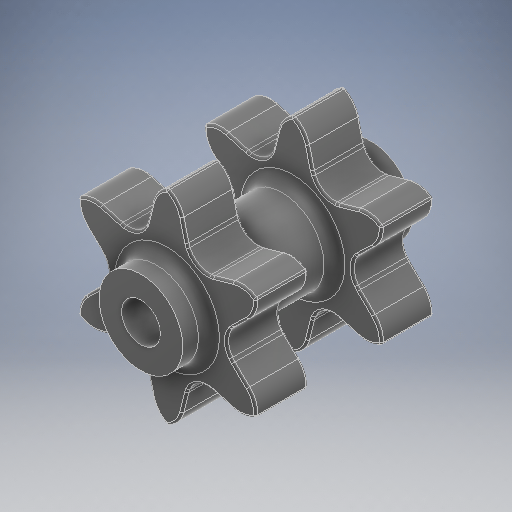
# Autodesk Inventor part: SprocketGeometry
Saved by Autodesk Inventor 2026.1 (Build 301233000, 233)
## iProperties
Created: 2025-09-26
Part Number: SprocketGeometry
Material: Plastic, Opaque Black
Document SubType Name: Modeling
Designer: Teddy
Density: 0.952 g/cm^3
Appearance: Smooth - Black
Author: Teddy
Autodesk Inventor part; units mm, degrees
ref_plane "YZ Plane" through (0, 0, 0) normal (1, 0, 0) x (0, 1, 0)
ref_plane "XZ Plane" through (0, 0, 0) normal (0, 1, 0) x (-1, 0, 0)
ref_plane "XY Plane" through (0, 0, 0) normal (0, 0, 1) x (1, 0, 0)
sketch "Sketch1" plane through (0, 0, 0) normal (0, 0, 1) x (1, 0, 0)
  line L0 (-9.7902, 3.5752) -> (-8.0084, 1.8545)
  spline S0 degree 3 poles (-10.7537, 6.0542) (-10.7758, 5.6696) (-10.7287, 5.2836) (-10.4774, 4.4609) (-10.2116, 4.004) (-9.833, 3.6171) (-9.8117, 3.596) (-9.7902, 3.5752) knots 0 0 0 0 0.414162 0.414162 0.967573 0.967573 1 1 1 1
  spline S1 degree 3 poles (-7.9913, 6.691) (-8.0201, 6.6992) (-8.049, 6.7071) (-8.5734, 6.8415) (-9.1019, 6.8432) (-9.9401, 6.6495) (-10.2979, 6.4973) (-10.6199, 6.2859) knots 0 0 0 0 0.032427 0.032427 0.585838 0.585838 1 1 1 1
  line L1 (-7.9913, 6.691) -> (-5.6103, 6.0082)
  arc A0 (-5.1715, 5.9227) -> (-2.5435, 7.44) centre (-4.8997, 8.4865) ccw
  spline S2 degree 3 poles (-10.7537, 6.0542) (-10.7533, 6.0604) (-10.7527, 6.0666) (-10.7469, 6.1132) (-10.7332, 6.1525) (-10.6948, 6.219) (-10.6676, 6.2505) (-10.6302, 6.2788) (-10.6251, 6.2824) (-10.6199, 6.2859) knots 0 0 0 0 0.066671 0.066671 0.5 0.5 0.933329 0.933329 1 1 1 1
  spline S3 degree 3 poles (-5.1715, 5.9227) (-5.1884, 5.9245) (-5.2052, 5.9265) (-5.3494, 5.9446) (-5.4802, 5.9714) (-5.6103, 6.0082) knots 0 0 0 0 0.115694 0.115694 1 1 1 1
  line L2 (-1.7989, 10.2662) -> (-2.3981, 7.8628)
  spline S4 degree 3 poles (-2.3981, 7.8628) (-2.4313, 7.7317) (-2.4735, 7.605) (-2.5299, 7.471) (-2.5366, 7.4555) (-2.5435, 7.44) knots 0 0 0 0 0.884306 0.884306 1 1 1 1
  spline S5 degree 3 poles (-0.1338, 12.34) (-0.4779, 12.1669) (-0.7886, 11.9332) (-1.3754, 11.3041) (-1.6382, 10.8456) (-1.784, 10.3242) (-1.7916, 10.2952) (-1.7989, 10.2662) knots 0 0 0 0 0.414162 0.414162 0.967573 0.967573 1 1 1 1
  spline S6 degree 3 poles (-0.1338, 12.34) (-0.1282, 12.3428) (-0.1225, 12.3454) (-0.0793, 12.3637) (-0.0384, 12.3715) (0.0384, 12.3715) (0.0793, 12.3637) (0.1225, 12.3454) (0.1282, 12.3428) (0.1338, 12.34) knots 0 0 0 0 0.066671 0.066671 0.5 0.5 0.933329 0.933329 1 1 1 1
  spline S7 degree 3 poles (1.7989, 10.2662) (1.7916, 10.2952) (1.784, 10.3242) (1.6382, 10.8456) (1.3754, 11.3041) (0.7886, 11.9332) (0.4779, 12.1669) (0.1338, 12.34) knots 0 0 0 0 0.032427 0.032427 0.585838 0.585838 1 1 1 1
  line L3 (1.7989, 10.2662) -> (2.3981, 7.8628)
  spline S8 degree 3 poles (2.5435, 7.44) (2.5366, 7.4555) (2.5299, 7.471) (2.4735, 7.605) (2.4313, 7.7317) (2.3981, 7.8628) knots 0 0 0 0 0.115694 0.115694 1 1 1 1
  arc A1 (2.5435, 7.44) -> (5.1715, 5.9227) centre (4.8997, 8.4865) ccw
  spline S9 degree 3 poles (5.6103, 6.0082) (5.4802, 5.9714) (5.3494, 5.9446) (5.2052, 5.9265) (5.1884, 5.9245) (5.1715, 5.9227) knots 0 0 0 0 0.884306 0.884306 1 1 1 1
  line L4 (7.9913, 6.691) -> (5.6103, 6.0082)
  spline S10 degree 3 poles (10.6199, 6.2859) (10.2979, 6.4973) (9.9401, 6.6495) (9.1019, 6.8432) (8.5734, 6.8415) (8.049, 6.7071) (8.0201, 6.6992) (7.9913, 6.691) knots 0 0 0 0 0.414162 0.414162 0.967573 0.967573 1 1 1 1
  spline S11 degree 3 poles (10.6199, 6.2859) (10.6251, 6.2824) (10.6302, 6.2788) (10.6676, 6.2505) (10.6948, 6.219) (10.7332, 6.1525) (10.7469, 6.1132) (10.7527, 6.0666) (10.7533, 6.0604) (10.7537, 6.0542) knots 0 0 0 0 0.066671 0.066671 0.5 0.5 0.933329 0.933329 1 1 1 1
  spline S12 degree 3 poles (9.7902, 3.5752) (9.8117, 3.596) (9.833, 3.6171) (10.2116, 4.004) (10.4774, 4.4609) (10.7287, 5.2836) (10.7758, 5.6696) (10.7537, 6.0542) knots 0 0 0 0 0.032427 0.032427 0.585838 0.585838 1 1 1 1
  line L5 (8.0084, 1.8545) -> (9.7902, 3.5752)
  spline S13 degree 3 poles (7.715, 1.5173) (7.725, 1.531) (7.7351, 1.5446) (7.8229, 1.6604) (7.9115, 1.7603) (8.0084, 1.8545) knots 0 0 0 0 0.115694 0.115694 1 1 1 1
  arc A2 (7.715, 1.5173) -> (7.715, -1.5173) centre (9.7993, 0) ccw
  spline S14 degree 3 poles (8.0084, -1.8545) (7.9115, -1.7603) (7.8229, -1.6604) (7.7351, -1.5446) (7.725, -1.531) (7.715, -1.5173) knots 0 0 0 0 0.884306 0.884306 1 1 1 1
  line L6 (9.7902, -3.5752) -> (8.0084, -1.8545)
  spline S15 degree 3 poles (10.7537, -6.0542) (10.7758, -5.6696) (10.7287, -5.2836) (10.4774, -4.4609) (10.2116, -4.004) (9.833, -3.6171) (9.8117, -3.596) (9.7902, -3.5752) knots 0 0 0 0 0.414162 0.414162 0.967573 0.967573 1 1 1 1
  spline S16 degree 3 poles (10.7537, -6.0542) (10.7533, -6.0604) (10.7527, -6.0666) (10.7469, -6.1132) (10.7332, -6.1525) (10.6948, -6.219) (10.6676, -6.2505) (10.6302, -6.2788) (10.6251, -6.2824) (10.6199, -6.2859) knots 0 0 0 0 0.066671 0.066671 0.5 0.5 0.933329 0.933329 1 1 1 1
  spline S17 degree 3 poles (7.9913, -6.691) (8.0201, -6.6992) (8.049, -6.7071) (8.5734, -6.8415) (9.1019, -6.8432) (9.9401, -6.6495) (10.2979, -6.4973) (10.6199, -6.2859) knots 0 0 0 0 0.032427 0.032427 0.585838 0.585838 1 1 1 1
  line L7 (7.9913, -6.691) -> (5.6103, -6.0082)
  spline S18 degree 3 poles (5.1715, -5.9227) (5.1884, -5.9245) (5.2052, -5.9265) (5.3494, -5.9446) (5.4802, -5.9714) (5.6103, -6.0082) knots 0 0 0 0 0.115694 0.115694 1 1 1 1
  arc A3 (5.1715, -5.9227) -> (2.5435, -7.44) centre (4.8997, -8.4865) ccw
  spline S19 degree 3 poles (2.3981, -7.8628) (2.4313, -7.7317) (2.4735, -7.605) (2.5299, -7.471) (2.5366, -7.4555) (2.5435, -7.44) knots 0 0 0 0 0.884306 0.884306 1 1 1 1
  line L8 (1.7989, -10.2662) -> (2.3981, -7.8628)
  spline S20 degree 3 poles (0.1338, -12.34) (0.4779, -12.1669) (0.7886, -11.9332) (1.3754, -11.3041) (1.6382, -10.8456) (1.784, -10.3242) (1.7916, -10.2952) (1.7989, -10.2662) knots 0 0 0 0 0.414162 0.414162 0.967573 0.967573 1 1 1 1
  spline S21 degree 3 poles (0.1338, -12.34) (0.1282, -12.3428) (0.1225, -12.3454) (0.0793, -12.3637) (0.0384, -12.3715) (-0.0384, -12.3715) (-0.0793, -12.3637) (-0.1225, -12.3454) (-0.1282, -12.3428) (-0.1338, -12.34) knots 0 0 0 0 0.066671 0.066671 0.5 0.5 0.933329 0.933329 1 1 1 1
  spline S22 degree 3 poles (-1.7989, -10.2662) (-1.7916, -10.2952) (-1.784, -10.3242) (-1.6382, -10.8456) (-1.3754, -11.3041) (-0.7886, -11.9332) (-0.4779, -12.1669) (-0.1338, -12.34) knots 0 0 0 0 0.032427 0.032427 0.585838 0.585838 1 1 1 1
  line L9 (-1.7989, -10.2662) -> (-2.3981, -7.8628)
  spline S23 degree 3 poles (-2.5435, -7.44) (-2.5366, -7.4555) (-2.5299, -7.471) (-2.4735, -7.605) (-2.4313, -7.7317) (-2.3981, -7.8628) knots 0 0 0 0 0.115694 0.115694 1 1 1 1
  arc A4 (-2.5435, -7.44) -> (-5.1715, -5.9227) centre (-4.8997, -8.4865) ccw
  spline S24 degree 3 poles (-5.6103, -6.0082) (-5.4802, -5.9714) (-5.3494, -5.9446) (-5.2052, -5.9265) (-5.1884, -5.9245) (-5.1715, -5.9227) knots 0 0 0 0 0.884306 0.884306 1 1 1 1
  line L10 (-7.9913, -6.691) -> (-5.6103, -6.0082)
  spline S25 degree 3 poles (-10.6199, -6.2859) (-10.2979, -6.4973) (-9.9401, -6.6495) (-9.1019, -6.8432) (-8.5734, -6.8415) (-8.049, -6.7071) (-8.0201, -6.6992) (-7.9913, -6.691) knots 0 0 0 0 0.414162 0.414162 0.967573 0.967573 1 1 1 1
  spline S26 degree 3 poles (-10.6199, -6.2859) (-10.6251, -6.2824) (-10.6302, -6.2788) (-10.6676, -6.2505) (-10.6948, -6.219) (-10.7332, -6.1525) (-10.7469, -6.1132) (-10.7527, -6.0666) (-10.7533, -6.0604) (-10.7537, -6.0542) knots 0 0 0 0 0.066671 0.066671 0.5 0.5 0.933329 0.933329 1 1 1 1
  spline S27 degree 3 poles (-9.7902, -3.5752) (-9.8117, -3.596) (-9.833, -3.6171) (-10.2116, -4.004) (-10.4774, -4.4609) (-10.7287, -5.2836) (-10.7758, -5.6696) (-10.7537, -6.0542) knots 0 0 0 0 0.032427 0.032427 0.585838 0.585838 1 1 1 1
  line L11 (-8.0084, -1.8545) -> (-9.7902, -3.5752)
  arc A5 (-7.715, -1.5173) -> (-7.715, 1.5173) centre (-9.7993, 0) ccw
  spline S28 degree 3 poles (-7.715, -1.5173) (-7.725, -1.531) (-7.7351, -1.5446) (-7.8229, -1.6604) (-7.9115, -1.7603) (-8.0084, -1.8545) knots 0 0 0 0 0.115694 0.115694 1 1 1 1
  spline S29 degree 3 poles (-8.0084, 1.8545) (-7.9115, 1.7603) (-7.8229, 1.6604) (-7.7351, 1.5446) (-7.725, 1.531) (-7.715, 1.5173) knots 0 0 0 0 0.884306 0.884306 1 1 1 1
  point P0 (0, 0)
extrude "Extrusion1" add sketch "Sketch1" along normal mid plane 6.35
sketch "Sketch2" plane through (0, 0, 3.175) normal (0, 0, 1) x (1, 0, 0)
  line L0 (3.048, -3.302) -> (-3.048, -3.302) construction
  line L1 (-3.302, -3.048) -> (-3.302, 3.048) construction
  line L2 (-3.048, 3.302) -> (3.048, 3.302) construction
  line L3 (3.302, 3.048) -> (3.302, -3.048) construction
  line L4 (3.302, -3.302) -> (-3.302, 3.302) construction
  line L5 (-3.302, -3.302) -> (3.302, 3.302) construction
  arc A0 (-3.302, -3.048) -> (-3.048, -3.302) centre (-3.048, -3.048) ccw construction
  arc A1 (-3.048, 3.302) -> (-3.302, 3.048) centre (-3.048, 3.048) ccw construction
  arc A2 (3.302, 3.048) -> (3.048, 3.302) centre (3.048, 3.048) ccw construction
  arc A3 (3.048, -3.302) -> (3.302, -3.048) centre (3.048, -3.048) ccw construction
  circle A4 centre (0, 0) radius 2.3495
  circle A5 centre (0, 0) radius 5.08
  dimension "d2" = 6.604
  dimension "d3" = 6.604
  dimension "d4" = 0.254
  dimension "d5" = 4.699
  dimension "d6" = 10.16
  constraints: 12 end point, 8 point on circle, 8 point on line, 8 tangent, 6 centre point, 3 equal radius, 2 coincident, 2 midpoint, 2 parallel, 1 horizontal, 1 perpendicular
  measures "d2" distance of L4.end L5.end
  measures "d3" distance of L5.end L4.start
  measures "d4" radius of A0
  measures "d5" diameter of A4
  measures "d6" diameter of A5
extrude "Extrusion2" add sketch "Sketch2" along normal blind 8.89
sketch "Sketch3" plane through (0, 0, 12.065) normal (0, 0, 1) x (1, 0, 0)
  line L0 (-9.7902, 3.5752) -> (-8.0084, 1.8545) projected
  ellipse E0 centre (-9.017, 1.1629) end of major axis (-7.5138, 0.0679) minor radius 1.1817 (-7.715, 1.5173) -> (-8.0084, 1.8545) ccw projected
  arc A0 (-7.715, -1.5173) -> (-7.715, 1.5173) centre (-9.7993, 0) ccw projected
  spline S0 degree 3 poles (-7.715, -1.5173) (-7.725, -1.531) (-7.7351, -1.5446) (-7.8229, -1.6604) (-7.9115, -1.7603) (-8.0084, -1.8545) knots 0 0 0 0 0.115694 0.115694 1 1 1 1 projected
  line L1 (-8.0084, -1.8545) -> (-9.7902, -3.5752) projected
  spline S1 degree 3 poles (-9.7902, -3.5752) (-9.8117, -3.596) (-9.833, -3.6171) (-10.2116, -4.004) (-10.4774, -4.4609) (-10.7287, -5.2836) (-10.7758, -5.6696) (-10.7537, -6.0542) knots 0 0 0 0 0.032427 0.032427 0.585838 0.585838 1 1 1 1 projected
  spline S2 degree 3 poles (-10.7537, -6.0542) (-10.7533, -6.0604) (-10.7527, -6.0666) (-10.7469, -6.1132) (-10.7332, -6.1525) (-10.6948, -6.219) (-10.6676, -6.2505) (-10.6302, -6.2788) (-10.6251, -6.2824) (-10.6199, -6.2859) knots 0 0 0 0 0.066671 0.066671 0.5 0.5 0.933329 0.933329 1 1 1 1 projected
  spline S3 degree 3 poles (-10.6199, -6.2859) (-10.2979, -6.4973) (-9.9401, -6.6495) (-9.1019, -6.8432) (-8.5734, -6.8415) (-8.049, -6.7071) (-8.0201, -6.6992) (-7.9913, -6.691) knots 0 0 0 0 0.414162 0.414162 0.967573 0.967573 1 1 1 1 projected
  line L2 (-7.9913, -6.691) -> (-5.6103, -6.0082) projected
  ellipse E1 centre (-5.5156, -7.2275) end of major axis (-3.8157, -6.4732) minor radius 1.1817 (-5.1715, -5.9227) -> (-5.6103, -6.0082) ccw projected
  arc A1 (-2.5435, -7.44) -> (-5.1715, -5.9227) centre (-4.8997, -8.4865) ccw projected
  spline S4 degree 3 poles (-2.5435, -7.44) (-2.5366, -7.4555) (-2.5299, -7.471) (-2.4735, -7.605) (-2.4313, -7.7317) (-2.3981, -7.8628) knots 0 0 0 0 0.115694 0.115694 1 1 1 1 projected
  line L3 (-2.3981, -7.8628) -> (-1.7989, -10.2662) projected
  spline S5 degree 3 poles (-1.7989, -10.2662) (-1.7916, -10.2952) (-1.784, -10.3242) (-1.6382, -10.8456) (-1.3754, -11.3041) (-0.7886, -11.9332) (-0.4779, -12.1669) (-0.1338, -12.34) knots 0 0 0 0 0.032427 0.032427 0.585838 0.585838 1 1 1 1 projected
  spline S6 degree 3 poles (-0.1338, -12.34) (-0.1282, -12.3428) (-0.1225, -12.3454) (-0.0793, -12.3637) (-0.0384, -12.3715) (0.0384, -12.3715) (0.0793, -12.3637) (0.1225, -12.3454) (0.1282, -12.3428) (0.1338, -12.34) knots 0 0 0 0 0.066671 0.066671 0.5 0.5 0.933329 0.933329 1 1 1 1 projected
  spline S7 degree 3 poles (0.1338, -12.34) (0.4779, -12.1669) (0.7886, -11.9332) (1.3754, -11.3041) (1.6382, -10.8456) (1.784, -10.3242) (1.7916, -10.2952) (1.7989, -10.2662) knots 0 0 0 0 0.414162 0.414162 0.967573 0.967573 1 1 1 1 projected
  line L4 (1.7989, -10.2662) -> (2.3981, -7.8628) projected
  ellipse E2 centre (3.5014, -8.3904) end of major axis (3.6981, -6.5411) minor radius 1.1817 (2.5435, -7.44) -> (2.3981, -7.8628) ccw projected
  arc A2 (5.1715, -5.9227) -> (2.5435, -7.44) centre (4.8997, -8.4865) ccw projected
  spline S8 degree 3 poles (5.1715, -5.9227) (5.1884, -5.9245) (5.2052, -5.9265) (5.3494, -5.9446) (5.4802, -5.9714) (5.6103, -6.0082) knots 0 0 0 0 0.115694 0.115694 1 1 1 1 projected
  line L5 (5.6103, -6.0082) -> (7.9913, -6.691) projected
  spline S9 degree 3 poles (7.9913, -6.691) (8.0201, -6.6992) (8.049, -6.7071) (8.5734, -6.8415) (9.1019, -6.8432) (9.9401, -6.6495) (10.2979, -6.4973) (10.6199, -6.2859) knots 0 0 0 0 0.032427 0.032427 0.585838 0.585838 1 1 1 1 projected
  spline S10 degree 3 poles (10.6199, -6.2859) (10.6251, -6.2824) (10.6302, -6.2788) (10.6676, -6.2505) (10.6948, -6.219) (10.7332, -6.1525) (10.7469, -6.1132) (10.7527, -6.0666) (10.7533, -6.0604) (10.7537, -6.0542) knots 0 0 0 0 0.066671 0.066671 0.5 0.5 0.933329 0.933329 1 1 1 1 projected
  spline S11 degree 3 poles (10.7537, -6.0542) (10.7758, -5.6696) (10.7287, -5.2836) (10.4774, -4.4609) (10.2116, -4.004) (9.833, -3.6171) (9.8117, -3.596) (9.7902, -3.5752) knots 0 0 0 0 0.414162 0.414162 0.967573 0.967573 1 1 1 1 projected
  line L6 (9.7902, -3.5752) -> (8.0084, -1.8545) projected
  ellipse E3 centre (9.017, -1.1629) end of major axis (10.5202, -2.2578) minor radius 1.1817 (7.715, -1.5173) -> (8.0084, -1.8545) ccw projected
  arc A3 (7.715, 1.5173) -> (7.715, -1.5173) centre (9.7993, 0) ccw projected
  spline S12 degree 3 poles (7.715, 1.5173) (7.725, 1.531) (7.7351, 1.5446) (7.8229, 1.6604) (7.9115, 1.7603) (8.0084, 1.8545) knots 0 0 0 0 0.115694 0.115694 1 1 1 1 projected
  line L7 (8.0084, 1.8545) -> (9.7902, 3.5752) projected
  spline S13 degree 3 poles (9.7902, 3.5752) (9.8117, 3.596) (9.833, 3.6171) (10.2116, 4.004) (10.4774, 4.4609) (10.7287, 5.2836) (10.7758, 5.6696) (10.7537, 6.0542) knots 0 0 0 0 0.032427 0.032427 0.585838 0.585838 1 1 1 1 projected
  spline S14 degree 3 poles (10.7537, 6.0542) (10.7533, 6.0604) (10.7527, 6.0666) (10.7469, 6.1132) (10.7332, 6.1525) (10.6948, 6.219) (10.6676, 6.2505) (10.6302, 6.2788) (10.6251, 6.2824) (10.6199, 6.2859) knots 0 0 0 0 0.066671 0.066671 0.5 0.5 0.933329 0.933329 1 1 1 1 projected
  spline S15 degree 3 poles (10.6199, 6.2859) (10.2979, 6.4973) (9.9401, 6.6495) (9.1019, 6.8432) (8.5734, 6.8415) (8.049, 6.7071) (8.0201, 6.6992) (7.9913, 6.691) knots 0 0 0 0 0.414162 0.414162 0.967573 0.967573 1 1 1 1 projected
  line L8 (7.9913, 6.691) -> (5.6103, 6.0082) projected
  ellipse E4 centre (5.5156, 7.2275) end of major axis (7.2154, 7.9818) minor radius 1.1817 (5.1715, 5.9227) -> (5.6103, 6.0082) ccw projected
  arc A4 (2.5435, 7.44) -> (5.1715, 5.9227) centre (4.8997, 8.4865) ccw projected
  spline S16 degree 3 poles (2.5435, 7.44) (2.5366, 7.4555) (2.5299, 7.471) (2.4735, 7.605) (2.4313, 7.7317) (2.3981, 7.8628) knots 0 0 0 0 0.115694 0.115694 1 1 1 1 projected
  line L9 (2.3981, 7.8628) -> (1.7989, 10.2662) projected
  spline S17 degree 3 poles (1.7989, 10.2662) (1.7916, 10.2952) (1.784, 10.3242) (1.6382, 10.8456) (1.3754, 11.3041) (0.7886, 11.9332) (0.4779, 12.1669) (0.1338, 12.34) knots 0 0 0 0 0.032427 0.032427 0.585838 0.585838 1 1 1 1 projected
  spline S18 degree 3 poles (0.1338, 12.34) (0.1282, 12.3428) (0.1225, 12.3454) (0.0793, 12.3637) (0.0384, 12.3715) (-0.0384, 12.3715) (-0.0793, 12.3637) (-0.1225, 12.3454) (-0.1282, 12.3428) (-0.1338, 12.34) knots 0 0 0 0 0.066671 0.066671 0.5 0.5 0.933329 0.933329 1 1 1 1 projected
  spline S19 degree 3 poles (-0.1338, 12.34) (-0.4779, 12.1669) (-0.7886, 11.9332) (-1.3754, 11.3041) (-1.6382, 10.8456) (-1.784, 10.3242) (-1.7916, 10.2952) (-1.7989, 10.2662) knots 0 0 0 0 0.414162 0.414162 0.967573 0.967573 1 1 1 1 projected
  line L10 (-1.7989, 10.2662) -> (-2.3981, 7.8628) projected
  ellipse E5 centre (-3.5014, 8.3904) end of major axis (-3.3047, 10.2396) minor radius 1.1817 (-2.5435, 7.44) -> (-2.3981, 7.8628) ccw projected
  arc A5 (-5.1715, 5.9227) -> (-2.5435, 7.44) centre (-4.8997, 8.4865) ccw projected
  spline S20 degree 3 poles (-5.1715, 5.9227) (-5.1884, 5.9245) (-5.2052, 5.9265) (-5.3494, 5.9446) (-5.4802, 5.9714) (-5.6103, 6.0082) knots 0 0 0 0 0.115694 0.115694 1 1 1 1 projected
  line L11 (-5.6103, 6.0082) -> (-7.9913, 6.691) projected
  spline S21 degree 3 poles (-7.9913, 6.691) (-8.0201, 6.6992) (-8.049, 6.7071) (-8.5734, 6.8415) (-9.1019, 6.8432) (-9.9401, 6.6495) (-10.2979, 6.4973) (-10.6199, 6.2859) knots 0 0 0 0 0.032427 0.032427 0.585838 0.585838 1 1 1 1 projected
  spline S22 degree 3 poles (-10.6199, 6.2859) (-10.6251, 6.2824) (-10.6302, 6.2788) (-10.6676, 6.2505) (-10.6948, 6.219) (-10.7332, 6.1525) (-10.7469, 6.1132) (-10.7527, 6.0666) (-10.7533, 6.0604) (-10.7537, 6.0542) knots 0 0 0 0 0.066671 0.066671 0.5 0.5 0.933329 0.933329 1 1 1 1 projected
  spline S23 degree 3 poles (-10.7537, 6.0542) (-10.7758, 5.6696) (-10.7287, 5.2836) (-10.4774, 4.4609) (-10.2116, 4.004) (-9.833, 3.6171) (-9.8117, 3.596) (-9.7902, 3.5752) knots 0 0 0 0 0.414162 0.414162 0.967573 0.967573 1 1 1 1 projected
  circle A6 centre (0, 0) radius 5.08 projected
  circle A7 centre (0, 0) radius 2.3495 projected
  constraints: 2 horizontal alignment, 28 other
extrude "Extrusion3" add sketch "Sketch3" along normal blind 6.35 contours S23 S22 S21 L11 S20 A5 E5 L10 S19 S18 S17 L9 S16 A4 E4 L8 S15 S14 S13 L7 S12 A3 E3 L6 S11 S10 S9 L5 S8 A2 E2 L4 S7 S6 S5 L3 S4 A1 E1 L2 S3 S2 S1 L1 S0 A0 E0 L0 | A6
sketch "Sketch4" plane through (0, 0, 18.415) normal (0, 0, 1) x (1, 0, 0)
  circle A0 centre (0, 0) radius 2.3495 projected
  circle A1 centre (0, 0) radius 5.08 projected
extrude "Extrusion4" add sketch "Sketch4" along normal blind 3.175
sketch "Sketch5" plane through (0, 0, 21.59) normal (0, 0, 1) x (1, 0, 0)
  circle A0 centre (0, 0) radius 2.3495 projected
extrude "Extrusion5" cut sketch "Sketch5" against normal through all
sketch "Sketch6" plane through (0, 0, -3.175) normal (0, 0, -1) x (-1, 0, 0)
  circle A0 centre (0, 0) radius 5.08 projected
  circle A1 centre (0, 0) radius 2.3495 projected
extrude "Extrusion6" add sketch "Sketch6" along normal blind 3.175
fillet "Fillet1" radius 1.27 4 edges at (-5.08, 0, 3.175) (5.08, 0, -3.175) (-5.08, 0, 12.065) (-5.08, 0, 18.415)
fillet "Fillet2" radius 0.254 192 edges at (-6.8008, 6.3496, 12.065) (-5.3896, 5.9555, 12.065) (-3.6106, 6.2538, 12.065) (-2.4627, 7.6456, 12.065) (-2.0985, 9.0645, 12.065) (-1.1905, 11.4896, 12.065) (0, 12.3715, 12.065) (1.1905, 11.4896, 12.065) (2.0985, 9.0645, 12.065) (2.4628, 7.6453, 12.065) (3.6106, 6.2538, 12.065) (5.3899, 5.9556, 12.065) (6.8008, 6.3496, 12.065) (9.355, 6.7758, 12.065) (10.714, 6.1858, 12.065) (10.5456, 4.7138, 12.065) (8.8993, 2.7149, 12.065) (7.8525, 1.6898, 12.065) (7.2212, 0, 12.065) (7.8526, -1.69, 12.065) (8.8993, -2.7149, 12.065) (10.5456, -4.7138, 12.065) (10.714, -6.1858, 12.065) (9.355, -6.7758, 12.065) (6.8008, -6.3496, 12.065) (5.3896, -5.9555, 12.065) (3.6106, -6.2538, 12.065) (2.4627, -7.6456, 12.065) (2.0985, -9.0645, 12.065) (1.1905, -11.4896, 12.065) (0, -12.3715, 12.065) (-1.1905, -11.4896, 12.065) (-2.0985, -9.0645, 12.065) (-2.4628, -7.6453, 12.065) (-3.6106, -6.2538, 12.065) (-5.3899, -5.9556, 12.065) (-6.8008, -6.3496, 12.065) (-9.355, -6.7758, 12.065) (-10.714, -6.1858, 12.065) (-10.5456, -4.7138, 12.065) (-8.8993, -2.7149, 12.065) (-7.8525, -1.6898, 12.065) (-7.2212, 0, 12.065) (-7.8526, 1.69, 12.065) (-8.8993, 2.7149, 12.065) (-10.5456, 4.7138, 12.065) (-10.714, 6.1858, 12.065) (-9.355, 6.7758, 12.065) (-8.8993, 2.7149, 3.175) (-7.8525, 1.6898, 3.175) (-7.2212, 0, 3.175) (-7.8525, -1.6898, 3.175) (-8.8993, -2.7149, 3.175) (-10.5456, -4.7138, 3.175) (-10.714, -6.1858, 3.175) (-9.355, -6.7758, 3.175) (-6.8008, -6.3496, 3.175) (-5.3896, -5.9555, 3.175) (-3.6106, -6.2538, 3.175) (-2.4628, -7.6453, 3.175) (-2.0985, -9.0645, 3.175) (-1.1905, -11.4896, 3.175) (0, -12.3715, 3.175) (1.1905, -11.4896, 3.175) (2.0985, -9.0645, 3.175) (2.4628, -7.6453, 3.175) (3.6106, -6.2538, 3.175) (5.3896, -5.9555, 3.175) (6.8008, -6.3496, 3.175) (9.355, -6.7758, 3.175) (10.714, -6.1858, 3.175) (10.5456, -4.7138, 3.175) (8.8993, -2.7149, 3.175) (7.8525, -1.6898, 3.175) (7.2212, 0, 3.175) (7.8525, 1.6898, 3.175) (8.8993, 2.7149, 3.175) (10.5456, 4.7138, 3.175) (10.714, 6.1858, 3.175) (9.355, 6.7758, 3.175) (6.8008, 6.3496, 3.175) (5.3896, 5.9555, 3.175) (3.6106, 6.2538, 3.175) (2.4628, 7.6453, 3.175) (2.0985, 9.0645, 3.175) (1.1905, 11.4896, 3.175) (0, 12.3715, 3.175) (-1.1905, 11.4896, 3.175) (-2.0985, 9.0645, 3.175) (-2.4628, 7.6453, 3.175) (-3.6106, 6.2538, 3.175) (-5.3896, 5.9555, 3.175) (-6.8008, 6.3496, 3.175) (-9.355, 6.7758, 3.175) (-10.714, 6.1858, 3.175) (-10.5456, 4.7138, 3.175) (-6.8008, 6.3496, 18.415) (-9.355, 6.7758, 18.415) (-10.714, 6.1858, 18.415) (-10.5456, 4.7138, 18.415) (-8.8993, 2.7149, 18.415) (-7.8526, 1.69, 18.415) (-7.2212, 0, 18.415) (-7.8525, -1.6898, 18.415) (-8.8993, -2.7149, 18.415) (-10.5456, -4.7138, 18.415) (-10.714, -6.1858, 18.415) (-9.355, -6.7758, 18.415) (-6.8008, -6.3496, 18.415) (-5.3899, -5.9556, 18.415) (-3.6106, -6.2538, 18.415) (-2.4628, -7.6453, 18.415) (-2.0985, -9.0645, 18.415) (-1.1905, -11.4896, 18.415) (0, -12.3715, 18.415) (1.1905, -11.4896, 18.415) (2.0985, -9.0645, 18.415) (2.4627, -7.6456, 18.415) (3.6106, -6.2538, 18.415) (5.3896, -5.9555, 18.415) (6.8008, -6.3496, 18.415) (9.355, -6.7758, 18.415) (10.714, -6.1858, 18.415) (10.5456, -4.7138, 18.415) (8.8993, -2.7149, 18.415) (7.8526, -1.69, 18.415) (7.2212, 0, 18.415) (7.8525, 1.6898, 18.415) (8.8993, 2.7149, 18.415) (10.5456, 4.7138, 18.415) (10.714, 6.1858, 18.415) (9.355, 6.7758, 18.415) (6.8008, 6.3496, 18.415) (5.3899, 5.9556, 18.415) (3.6106, 6.2538, 18.415) (2.4628, 7.6453, 18.415) (2.0985, 9.0645, 18.415) (1.1905, 11.4896, 18.415) (0, 12.3715, 18.415) (-1.1905, 11.4896, 18.415) (-2.0985, 9.0645, 18.415) (-2.4627, 7.6456, 18.415) (-3.6106, 6.2538, 18.415) (-5.3896, 5.9555, 18.415) (-8.8993, 2.7149, -3.175) (-10.5456, 4.7138, -3.175) (-10.714, 6.1858, -3.175) (-9.355, 6.7758, -3.175) (-6.8008, 6.3496, -3.175) (-5.3896, 5.9555, -3.175) (-3.6106, 6.2538, -3.175) (-2.4628, 7.6453, -3.175) (-2.0985, 9.0645, -3.175) (-1.1905, 11.4896, -3.175) (0, 12.3715, -3.175) (1.1905, 11.4896, -3.175) (2.0985, 9.0645, -3.175) (2.4628, 7.6453, -3.175) (3.6106, 6.2538, -3.175) (5.3896, 5.9555, -3.175) (6.8008, 6.3496, -3.175) (9.355, 6.7758, -3.175) (10.714, 6.1858, -3.175) (10.5456, 4.7138, -3.175) (8.8993, 2.7149, -3.175) (7.8525, 1.6898, -3.175) (7.2212, 0, -3.175) (7.8525, -1.6898, -3.175) (8.8993, -2.7149, -3.175) (10.5456, -4.7138, -3.175) (10.714, -6.1858, -3.175) (9.355, -6.7758, -3.175) (6.8008, -6.3496, -3.175) (5.3896, -5.9555, -3.175) (3.6106, -6.2538, -3.175) (2.4628, -7.6453, -3.175) (2.0985, -9.0645, -3.175) (1.1905, -11.4896, -3.175) (0, -12.3715, -3.175) (-1.1905, -11.4896, -3.175) (-2.0985, -9.0645, -3.175) (-2.4628, -7.6453, -3.175) (-3.6106, -6.2538, -3.175) (-5.3896, -5.9555, -3.175) (-6.8008, -6.3496, -3.175) (-9.355, -6.7758, -3.175) (-10.714, -6.1858, -3.175) (-10.5456, -4.7138, -3.175) (-8.8993, -2.7149, -3.175) (-7.8525, -1.6898, -3.175) (-7.2212, 0, -3.175) (-7.8525, 1.6898, -3.175)
body "Solid1"
